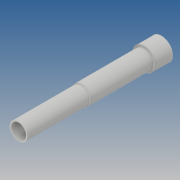
# Autodesk Inventor part: p1
Saved by Autodesk Inventor 2019 (Build 230136000, 136)
## iProperties
Created: 2019-03-23
Part Number: p1
Material: Générique
Document SubType Name: Modeling
Designer: Theo
Density: 1 g/cm^3
Appearance: Par défaut
Author: Theo
Autodesk Inventor part; units mm, degrees
ref_plane "YZ Plane" through (0, 0, 0) normal (1, 0, 0) x (0, 1, 0)
ref_plane "XZ Plane" through (0, 0, 0) normal (0, 1, 0) x (-1, 0, 0)
ref_plane "XY Plane" through (0, 0, 0) normal (0, 0, 1) x (1, 0, 0)
sketch "Esquisse1" plane through (0, 0, 0) normal (1, 0, 0) x (0, 1, 0)
  line L0 (0, 0) -> (0, 13.2431)
  line L1 (6, 11.3426) -> (6, 114)
  line L2 (6, 11.3426) -> (8, 0)
  line L3 (8, 0) -> (9, 0)
  line L4 (9, 0) -> (9, 14)
  line L5 (9, 14) -> (7.5, 14)
  line L6 (7.5, 14) -> (7.5, 64)
  line L7 (7, 64) -> (7, 114)
  line L8 (7, 64) -> (7.5, 64)
  line L9 (7, 114) -> (6, 114)
  dimension "d0" = 12
  dimension "d1" = 1
  dimension "d2" = 170
  dimension "d3" = 16
  dimension "d4" = 15
  dimension "d6" = 14
  dimension "d7" = 14
  dimension "d8" = 50
  dimension "d9" = 50
  constraints: 20 end point, 5 vertical, 4 horizontal, 1 horizontal alignment
  measures "d0" diameter of L1 L0
  measures "d1" distance of L2.end L3.end
  measures "d2" angle of L1 L2
  measures "d3" diameter of L2.end L0
  measures "d4" diameter of L6 L0
  measures "d6" distance between parallel lines of L5 L3
  measures "d7" diameter of L7 L0
  measures "d8" distance between parallel lines of L5 L8
  measures "d9" distance from line of L7.end L8
revolve "Révolution1" add sketch "Esquisse1" angle 360 about axis through (0, 0, 0) along (0, 0, 1)
